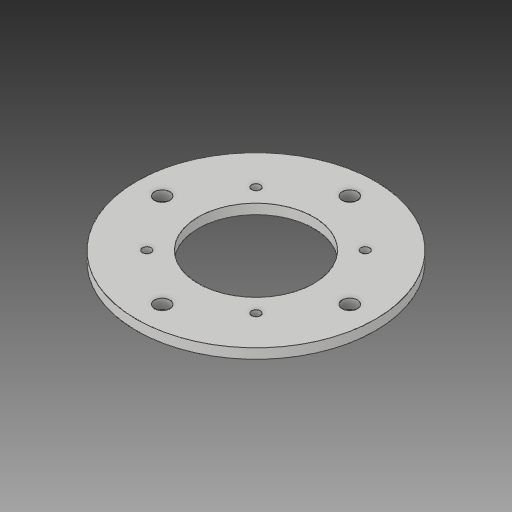
# Autodesk Inventor part: Servo Flange
Saved by Autodesk Inventor 2019 (Build 230136000, 136)
## iProperties
Created: 2017-12-22
Part Number: Servo Flange
Material: Generic
Document SubType Name: Modeling
Designer: torba
Density: 1 g/cm^3
Appearance: Default
Author: torba
Autodesk Inventor part; units mm, degrees
ref_plane "YZ Plane" through (0, 0, 0) normal (1, 0, 0) x (0, 1, 0)
ref_plane "XZ Plane" through (0, 0, 0) normal (0, 1, 0) x (-1, 0, 0)
ref_plane "XY Plane" through (0, 0, 0) normal (0, 0, 1) x (1, 0, 0)
sketch "Sketch1" plane through (0, 0, 0) normal (0, 1, 0) x (-1, 0, 0)
  line L0 (-6.5711, 78.1991) -> (-6.5711, 6.5711) construction
  arc A0 (0, 84.7702) -> (-6.5711, 78.1991) centre (0, 78.1991) ccw construction
  line L1 (71.628, 84.7702) -> (0, 84.7702) construction
  line L2 (-6.5711, 78.1991) -> (-6.5711, 6.5711) construction
  arc A1 (-6.5711, 6.5711) -> (0, 0) centre (0, 6.5711) ccw construction
  line L3 (0, 0) -> (71.628, 0) construction
  arc A2 (71.628, 0) -> (78.1991, 6.5711) centre (71.628, 6.5711) ccw construction
  line L4 (78.1991, 6.5711) -> (78.1991, 78.1991) construction
  arc A3 (78.1991, 78.1991) -> (71.628, 84.7702) centre (71.628, 78.1991) ccw construction
  line L5 (71.628, 84.7702) -> (0, 84.7702) construction
  arc A4 (0, 84.7702) -> (-6.5711, 78.1991) centre (0, 78.1991) ccw construction
  circle A5 centre (35.814, 42.3851) radius 36.7665
  circle A6 centre (70.6125, 77.1836) radius 3 construction
  circle A7 centre (1.0155, 77.1836) radius 3 construction
  circle A8 centre (17.6008, 80.7072) radius 3.875 construction
  circle A9 centre (-2.5081, 24.1719) radius 3.875 construction
  circle A10 centre (74.1361, 60.5983) radius 3.875 construction
  circle A11 centre (54.0272, 4.063) radius 3.875 construction
  circle A12 centre (1.0155, 7.5866) radius 3 construction
  circle A13 centre (70.6125, 7.5866) radius 3 construction
  line L6 (0, 85.77) -> (71.628, 85.77) construction
  arc A14 (0, 85.77) -> (-7.5709, 78.1991) centre (0, 78.1991) ccw construction
  line L7 (-7.5709, 6.5711) -> (-7.5709, 78.1991) construction
  arc A15 (-7.5709, 6.5711) -> (0, -0.9998) centre (0, 6.5711) ccw construction
  line L8 (71.628, -0.9998) -> (0, -0.9998) construction
  arc A16 (71.628, -0.9998) -> (79.1989, 6.5711) centre (71.628, 6.5711) ccw construction
  line L9 (79.1989, 78.1991) -> (79.1989, 6.5711) construction
  arc A17 (79.1989, 78.1991) -> (71.628, 85.77) centre (71.628, 78.1991) ccw construction
  circle A18 centre (35.814, 42.3851) radius 76.2
  line L10 (35.814, 150.1482) -> (143.5771, 42.3851) construction
  line L11 (143.5771, 42.3851) -> (35.814, -65.378) construction
  line L12 (35.814, -65.378) -> (-71.9491, 42.3851) construction
  line L13 (-71.9491, 42.3851) -> (35.814, 150.1482) construction
  line L14 (35.814, 150.1482) -> (35.814, -65.378) construction
  line L15 (143.5771, 42.3851) -> (-71.9491, 42.3851) construction
  line L16 (35.814, 150.1482) -> (188.214, 150.1482) construction
  line L17 (35.814, -33.8149) -> (35.814, -0.9998) construction
  line L18 (112.014, 42.3851) -> (79.1989, 42.3851) construction
  line L19 (35.814, 118.5851) -> (35.814, 85.77) construction
  line L20 (-40.386, 42.3851) -> (-7.5709, 42.3851) construction
  point P0 (86.7439, 21.4846)
  point P1 (-23.9785, 42.3851)
  point P2 (35.814, -17.4074)
  point P3 (95.6065, 42.3851)
  point P4 (35.814, 102.1776)
  point P5 (70.6125, 7.5866)
  dimension "d0" = 152.4
  dimension "d1" = 7.75
  dimension "d2" = 7.5709
  dimension "d3" = 6.5711
  dimension "d4" = 6
  dimension "d5" = 73.533
  dimension "d6" = 6.5711
  dimension "d7" = 90
  dimension "d8" = 90
  dimension "d9" = 85.77
  dimension "d10" = 85.77
  dimension "d11" = 79.1989
  dimension "d12" = 84.7702
  dimension "d13" = 84.7702
  dimension "d14" = 6.5711
  dimension "d15" = 7.5449
  dimension "d16" = 63.2856
  dimension "d17" = 5.0629
  dimension "d18" = 24.1719
  dimension "d19" = 7.5709
  dimension "d20" = 8.5865
  dimension "d21" = 7.5866
  dimension "d22" = 8.5865
  dimension "d23" = 77.1836
  dimension "d24" = 25.1717
  dimension "d25" = 80.7072
  dimension "d26" = 43.385
  dimension "d27" = 42.3851
  dimension "d28" = 61.5982
  dimension "d29" = 4.063
  dimension "d30" = 78.1834
  dimension "d31" = 7.5866
  dimension "d32" = 78.1834
  dimension "d33" = 77.1836
  dimension "d34" = 79.1989
  dimension "d35" = 79.1989
  dimension "d36" = 81.707
  dimension "d37" = 60.5983
  dimension "d38" = 78.1991
  dimension "d39" = 45
  dimension "d40" = 152.4
  dimension "d41" = 152.4
  constraints: 42 end point, 22 point on circle, 19 centre point, 16 tangent, 10 midpoint, 9 equal radius, 8 point on line, 7 parallel, 4 coincident, 4 concentric, 2 horizontal, 1 equal length, 1 perpendicular, 1 vertical
  measures "d0" diameter of A18
  measures "d1" diameter of A10
  measures "d2" radius of A17
  measures "d3" radius of A3
  measures "d4" diameter of A6
  measures "d5" diameter of A5
  measures "d6" radius of A0
  measures "d7" angle of L1 L9
  measures "d8" angle of L1 L0
  measures "d9" distance between parallel lines of L9 L2
  measures "d10" distance between parallel lines of L8 L5
  measures "d11" distance from line of point (0, 0) L9
  measures "d12" distance from line of point (0, 0) L1
  measures "d13" distance from line of point (0, 0) L5
  measures "d14" distance from line of point (0, 0) L0
  measures "d15" distance from line of point (86.744, 21.485) L9
  measures "d16" distance from line of point (86.744, 21.485) L1
  measures "d17" distance from line of A10.centre L9
  measures "d18" distance from line of A10.centre L1
  measures "d19" distance from line of L1.start L9
  measures "d20" distance from line of A6.centre L9
  measures "d21" distance from line of A6.centre L1
  measures "d22" distance from line of A13.centre L9
  measures "d23" distance from line of A13.centre L1
  measures "d24" distance from line of A11.centre L9
  measures "d25" distance from line of A11.centre L1
  measures "d26" distance from line of A5.centre L9
  measures "d27" distance from line of A5.centre L1
  measures "d28" distance from line of A8.centre L9
  measures "d29" distance from line of A8.centre L1
  measures "d30" distance from line of A7.centre L9
  measures "d31" distance from line of A7.centre L1
  measures "d32" distance from line of A12.centre L9
  measures "d33" distance from line of A12.centre L1
  measures "d34" distance from line of L1.end L9
  measures "d35" distance from line of A0.centre L9
  measures "d36" distance from line of A9.centre L9
  measures "d37" distance from line of A9.centre L1
  measures "d38" distance from line of L0.end L1
  measures "d39" angle of L10 L16
  measures "d40" distance of L10.end L11.end
  measures "d41" distance between parallel lines of L13 L11
extrude "Extrusion1" add sketch "Sketch1" along normal blind 6.35
hole "Hole1" at (-70.6125, 0, 77.1836) at (-70.6125, 0, 7.5866) at (-1.0155, 0, 7.5866) at (-1.0155, 0, 77.1836) direction (0, 1, 0) diameter 5.588 depth 6.5711 tip angle 118
hole "Hole2" at (23.9785, 0, 42.3851) at (-35.814, 0, -17.4074) at (-95.6065, 0, 42.3851) at (-35.814, 0, 102.1776) direction (0, 1, 0) diameter 9.8044 depth 6.5711 tip angle 118
equation "\"d49\" = d6"
equation "\"d56\" = d6"
body "Solid1"
